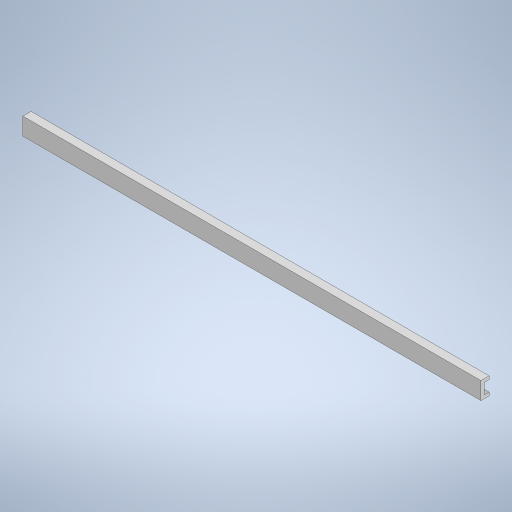
# Autodesk Inventor part: направляющая для стола
Saved by Autodesk Inventor 2023.1 (Build 271208000, 208)
## iProperties
Created: 2023-03-03
Part Number: направляющая для стола
Material: Типовые
Document SubType Name: Modeling
Designer: User
Density: 1 g/cm^3
Appearance: По умолчанию
Author: User
Autodesk Inventor part; units mm, degrees
ref_plane "YZ Plane" through (0, 0, 0) normal (1, 0, 0) x (0, 1, 0)
ref_plane "XZ Plane" through (0, 0, 0) normal (0, 1, 0) x (-1, 0, 0)
ref_plane "XY Plane" through (0, 0, 0) normal (0, 0, 1) x (1, 0, 0)
sketch "Эскиз1" plane through (0, 0, 0) normal (0, 0, 1) x (1, 0, 0)
  line L0 (-119.1026, 5.3) -> (20.8974, 5.3)
  line L1 (20.8974, 5.3) -> (20.8974, 0)
  line L2 (20.8974, 0) -> (-119.1026, 0)
  line L3 (-119.1026, 0) -> (-119.1026, 5.3)
  point P0 (0, 0)
  point P1 (20.8974, 2.65)
  dimension "d0" = 5.3
  dimension "d1" = 140
  constraints: 8 end point, 2 parallel, 1 horizontal, 1 horizontal alignment, 1 midpoint, 1 perpendicular
  measures "d0" distance between parallel lines of L0 L2
  measures "d1" distance from line of point (20.897, 2.65) L3
extrude "Выдавливание1" add sketch "Эскиз1" along normal blind 1
sketch "Эскиз2" plane through (0, 0, 0) normal (0, 0, -1) x (-1, 0, 0)
  line L0 (-20.8974, 5.3) -> (119.1026, 5.3) projected
  line L1 (119.1026, 0) -> (-20.8974, 0) projected
  line L2 (119.1026, 5.3) -> (119.1026, 0) projected
  line L3 (-20.8974, 5.3) -> (119.1026, 5.3) projected
  line L4 (-20.8974, 0) -> (-20.8974, 5.3) projected
  line L5 (-20.8974, 0) -> (-20.8974, 5.3) projected
  line L6 (119.1026, 5.3) -> (119.1026, 0) projected
  line L7 (-20.8974, 5.3) -> (119.1026, 5.3)
  line L8 (119.1026, 5.3) -> (119.1026, 4.3)
  line L9 (119.1026, 4.3) -> (-20.8974, 4.3)
  line L10 (-20.8974, 4.3) -> (-20.8974, 5.3)
  line L11 (119.1026, 0) -> (-20.8974, 0)
  line L12 (-20.8974, 0) -> (-20.8974, 1)
  line L13 (-20.8974, 1) -> (119.1026, 1)
  line L14 (119.1026, 1) -> (119.1026, 0)
  point P0 (0, 0)
  dimension "d4" = 1
  dimension "d5" = 1
  constraints: 16 end point, 4 parallel, 2 horizontal, 2 perpendicular, 2 point on line
  measures "d4" distance between parallel lines of L0 L9
  measures "d5" distance between parallel lines of L13 L1
extrude "Выдавливание2" add sketch "Эскиз2" along normal blind 1.5 contours L0 L2 L9 L4 | L13 L2 L1 L4
